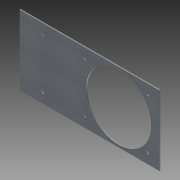
# Autodesk Inventor part: Fore_Base
Saved by Autodesk Inventor 2011 SP1 (Build 150282100, 282)
## iProperties
Created: 2011-05-30
Part Number: Fore_Base
Document SubType Name: Modeling
Designer: Andrew G. Meyer
Mass: 218.11 g
Surface Area: 1443.28 cm^2
Volume: 218.11 cm^3
Density: 1 g/cm^3
Author: Andrew G. Meyer
Autodesk Inventor part; units mm, degrees
ref_plane "YZ Plane" through (0, 0, 0) normal (1, 0, 0) x (0, 1, 0)
ref_plane "XZ Plane" through (0, 0, 0) normal (0, 1, 0) x (-1, 0, 0)
ref_plane "XY Plane" through (0, 0, 0) normal (0, 0, 1) x (1, 0, 0)
sketch "Sketch1" plane through (0, 0, 0) normal (0, 0, 1) x (1, 0, 0)
  line L0 (-139.7, 114.3) -> (317.5, 114.3)
  line L1 (317.5, 114.3) -> (317.5, -114.3)
  line L2 (317.5, -114.3) -> (-139.7, -114.3)
  line L3 (-139.7, -114.3) -> (-139.7, 114.3)
  point P0 (0, 0)
  dimension "d0" = 457.2
  dimension "d1" = 228.6
  dimension "d2" = 114.3
  dimension "d3" = 139.7
  constraints: 8 end point, 2 parallel, 1 horizontal, 1 perpendicular
  measures "d0" distance of L0.start L0.end
  measures "d1" distance of L2.end L0.start
  measures "d2" distance from line of L0 point (0, 0)
  measures "d3" distance from line of L3 point (0, 0)
extrude "Extrusion1" add sketch "Sketch1" against normal blind 3.175
hole "Hole1" at (184.15, 0, 0) direction (0, 0, -1) diameter 212.725 depth 25.4 tip angle 118
hole "Hole2" at (-63.5, 82.55, 0) direction (0, 0, -1) diameter 7.9375 depth 25.4 tip angle 118
hole "Hole3" at (-63.5, -82.55, 0) direction (0, 0, -1) diameter 7.9375 depth 25.4 tip angle 118
hole "Hole4" at (73.025, 82.55, 0) direction (0, 0, -1) diameter 7.9375 depth 25.4 tip angle 118
hole "Hole5" at (73.025, -82.55, 0) direction (0, 0, -1) diameter 6.35 depth 25.4 tip angle 118
hole "Hole6" at (279.4, 82.55, 0) direction (0, 0, -1) diameter 7.9375 depth 25.4 tip angle 118
hole "Hole7" at (279.4, -82.55, 0) direction (0, 0, -1) diameter 7.9375 depth 25.4 tip angle 118
body "Solid1"
